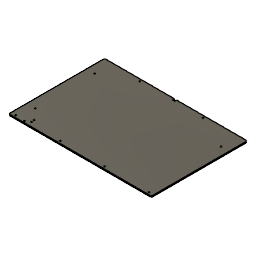
SolidBackPlate (Autodesk Fusion 360 design; units mm, degrees)
part number: 2026-09-01-01-20-22-232
part number: 2026-09-01-01-20-22-711
Autodesk Fusion 360 part; units mm, degrees
sketch "Cut_Profile_1to1_QTY1" plane through (0, 0, 0) normal (0, 0, 1) x (1, 0, 0) in component "SolidBackPlate"
  line L0 (-178.5, -122) -> (178.5, -122)
  arc A0 (178.5, -122) -> (181.5, -119) centre (178.5, -119) ccw
  line L1 (181.5, -119) -> (181.5, 119)
  arc A1 (181.5, 119) -> (178.5, 122) centre (178.5, 119) ccw
  line L2 (178.5, 122) -> (1.5, 122)
  line L3 (1.5, 122) -> (1.5, 117)
  line L4 (1.5, 117) -> (-3.5, 117)
  line L5 (-3.5, 117) -> (-3.5, 122)
  line L6 (-3.5, 122) -> (-178.5, 122)
  arc A2 (-178.5, 122) -> (-181.5, 119) centre (-178.5, 119) ccw
  line L7 (-181.5, 119) -> (-181.5, -119)
  arc A3 (-181.5, -119) -> (-178.5, -122) centre (-178.5, -119) ccw
  circle A4 centre (-86.5, 116) radius 1.6
  circle A5 centre (74.5, 116) radius 1.6
  circle A6 centre (-160.5, 76) radius 1.6
  circle A7 centre (160.5, 76) radius 1.6
  circle A8 centre (-169.5, -116) radius 1.6
  circle A9 centre (-56.5, -116) radius 1.6
  circle A10 centre (56.5, -116) radius 1.6
  circle A11 centre (169.5, -116) radius 1.6
  circle A12 centre (-145.5, -118) radius 1.6
  circle A13 centre (-134.5, -111) radius 1.6
  circle A14 centre (-135.5, -103) radius 1.6
  circle A15 centre (-159.5, -76) radius 1.6
extrude "Acrylic_Plate_3mm" add sketch "Cut_Profile_1to1_QTY1" along normal blind 3 in component "SolidBackPlate"
component "SolidBackPlate" placed x (1, 0, 0) y (0, 1, 0) z (0, 0, 1) at (0, 0, 0)
equation "mainboardLength = 355.0 mm" comment "Motherboard envelope length"
equation "mainboardWidth = 236.0 mm" comment "Motherboard envelope width"
equation "acrylicThickness = 3.0 mm" comment "Acrylic sheet thickness"
equation "assemblyClearance = 1.0 mm" comment "Clearance reserved around the motherboard"
equation "sideWallThickness = 3.0000000000000004 mm" comment "Original side-wall allowance retained in plate size"
equation "plateLength = mainboardLength + 2 * ( assemblyClearance + sideWallThickness )" comment "Finished plate length"
equation "plateWidth = mainboardWidth + 2 * ( assemblyClearance + sideWallThickness )" comment "Finished plate width"
equation "cornerRadius = 3.0000000000000004 mm" comment "Outside corner radius"
equation "mountHoleDiameter = 3.2000000000000006 mm" comment "M3 screw clearance-hole diameter"
equation "topNotchWidth = 5.0 mm" comment "Top-edge notch width"
equation "topNotchDepth = 5.0 mm" comment "Top-edge notch depth"
equation "topNotchRightEdgeOffsetRight = 180.0 mm" comment "Notch right edge from right plate edge"
equation "topMountOffsetSide = 21.0 mm" comment "Top mount centers from left/right plate edges"
equation "topMountOffsetTop = 46.00000000000000 mm" comment "Top mount centers from top plate edge"
equation "newTopHoleOffsetTop = 6.0 mm" comment "New M3 hole centers from top plate edge"
equation "newTopHole1OffsetLeft = 95.0 mm" comment "New left M3 hole center from left plate edge"
equation "newTopHole2OffsetRight = 107.0 mm" comment "New right M3 hole center from right plate edge"
equation "bottomMountOffsetLeft = 12.0 mm" comment "Leftmost bottom mount center from the left plate edge"
equation "bottomMountOffsetRight = 12.0 mm" comment "Rightmost bottom mount center from the right plate edge"
equation "bottomMountOffsetBottom = 6.0 mm" comment "Four bottom mount centers from bottom plate edge"
equation "bottomMountSpacing = ( plateLength - bottomMountOffsetLeft - bottomMountOffsetRight ) / 3" comment "Equal spacing between the four bottom mounts"
equation "additionalHole1Left = 36.0 mm" comment "Additional M3 hole 1 center from left plate edge"
equation "additionalHole1Bottom = 4.0 mm" comment "Additional M3 hole 1 center from bottom plate edge"
equation "additionalHole2Left = 47.0 mm" comment "Additional M3 hole 2 center from left plate edge"
equation "additionalHole2Bottom = 11.0 mm" comment "Additional M3 hole 2 center from bottom plate edge"
equation "additionalHole3Left = 46.00000000000000 mm" comment "Additional M3 hole 3 center from left plate edge"
equation "additionalHole3Bottom = 19.0 mm" comment "Additional M3 hole 3 center from bottom plate edge"
equation "additionalHole4Left = 22.0 mm" comment "Additional M3 hole 4 center from left plate edge"
equation "additionalHole4Bottom = 46.00000000000000 mm" comment "Additional M3 hole 4 center from bottom plate edge"
equation "cutQuantity = 1" comment "Cut one solid back plate"
equation "d31 = acrylicThickness"
named bodies: "SolidBackPlate_QTY1"
